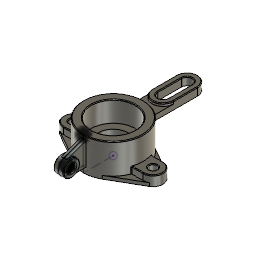
hw1 (Autodesk Fusion 360 design; units mm, degrees)
part number: 2026-08-05-10-36-34-167
Autodesk Fusion 360 part; units mm, degrees
sketch "스케치1" plane through (0, 0, 0) normal (0, 0, 1) x (1, 0, 0)
  circle A0 centre (0, 0) radius 45
  circle A1 centre (0, 0) radius 33
  circle A2 centre (0, 0) radius 22
  dimension "d3" = 90
  dimension "d9" = 66
  dimension "d10" = 44
  constraint concentric A0 A1
  constraint concentric A0 A2
  constraint coincident A0.centre A1.centre
  measures "d3" diameter of A0
  measures "d9" diameter of A1
  measures "d10" diameter of A2
sketch "스케치2" plane through (0, 0, 0) normal (0, 0, 1) x (1, 0, 0)
  line L0 (-8, 111) -> (-8, 75)
  arc A0 (-8, 75) -> (8, 75) centre (0, 75) ccw
  line L1 (8, 75) -> (8, 111)
  arc A1 (8, 111) -> (-8, 111) centre (0, 111) ccw
  line L2 (0, 111) -> (0, 75) construction
  line L3 (-16, 111) -> (-16, 75)
  arc A2 (-16, 75) -> (16, 75) centre (0, 75) ccw
  line L4 (16, 75) -> (16, 111)
  arc A3 (16, 111) -> (-16, 111) centre (0, 111) ccw
  line L5 (0, 111) -> (0, 75) construction
  line L6 (-16, 75) -> (-16, 42.0595)
  line L7 (16, 75) -> (16, 42.0595)
  circle A4 centre (0, 0) radius 45
  line L8 (0, 0) -> (0, 127) construction
  dimension "d15" = 16
  dimension "d16" = 32
  dimension "d17" = 36
  dimension "d18" = 75
  constraint tangent L0 A0
  constraint tangent A0 L1
  constraint parallel L0 L1
  constraint tangent L1 A1
  constraint tangent L0 A1
  constraint vertical L2
  constraint tangent L3 A2
  constraint tangent A2 L4
  constraint parallel L3 L4
  constraint tangent L4 A3
  constraint tangent L3 A3
  constraint parallel L1 L5
  constraint coincident A1.centre L2.start
  constraint coincident A0.centre L2.end
  constraint tangent A2 L6
  constraint tangent A2 L7
  constraint coincident L6.end A4
  constraint coincident L7.end A4
  constraint coincident A4.centre L8.start
  constraint midpoint A3 L8.end
  constraint vertical L8
  measures "d15" diameter of A0
  measures "d16" diameter of A2
  measures "d17" distance of A1.centre A0.centre
  measures "d18" distance of A0.centre A4.centre
extrude "돌출3" add sketch "스케치1" along normal blind 50 contours A0 makes body 1
extrude "돌출4" add sketch "스케치1" along normal blind 19 contours A1 bodies 1
extrude "돌출5" add sketch "스케치2" along normal blind 42 separate body contours L3 A2 L4 A3 makes body 2
extrude "돌출6" add sketch "스케치2" along normal blind 38 contours A2 L6 L7 A4 bodies 1 2
sketch "스케치3" plane through (0, 0, 0) normal (0, 0, 1) x (1, 0, 0)
  line L0 (-26, 36.7287) -> (-26, 127)
  line L1 (-26, 127) -> (26, 127)
  line L2 (26, 127) -> (26, 36.7287)
  circle A0 centre (0, 0) radius 45
  arc A1 (16, 111) -> (-16, 111) centre (0, 111) ccw
  line L3 (-16, 75) -> (-16, 42.0595)
  line L4 (16, 75) -> (16, 111)
  dimension "d26" = 10
  dimension "d27" = 10
  constraint vertical L0
  constraint perpendicular L0 L1
  constraint coincident L0.start A0
  constraint coincident L2.end A0
  constraint vertical L2
  constraint tangent L1 A1
  measures "d26" distance of L0 L3
  measures "d27" distance of L2 L4
extrude "돌출7" cut sketch "스케치3" along normal blind 30 contours L0 L1 L2 A0 bodies 1
sketch "스케치4" plane through (0, 0, 0) normal (0, 0, 1) x (1, 0, 0)
  line L0 (0, 0) -> (75, 0) construction
  circle A0 centre (60, 0) radius 6
  line L1 (42.4264, -15) -> (60, -15)
  line L2 (60, 15) -> (42.4264, 15)
  line L3 (60, -15) -> (60, 15) construction
  circle A1 centre (0, 0) radius 45
  arc A2 (60, -15) -> (60, 15) centre (60, 0) ccw
  line L4 (22.5, 38.9711) -> (67.5, 12.9904)
  line L5 (22.5, -38.9711) -> (67.5, -12.9904)
  dimension "d28" = 30
  dimension "d29" = 12
  dimension "d30" = 60
  constraint coincident L0.start A1.centre
  constraint horizontal L0
  constraint coincident A0.centre L0
  constraint coincident A0.centre A2.centre
  constraint horizontal L2
  constraint horizontal L1
  constraint coincident L1.end A2
  constraint coincident L2.start A2
  constraint perpendicular L0 L3
  constraint coincident A0.centre L3
  constraint coincident L1.end L3.start
  constraint coincident L2.start L3.end
  constraint coincident L2.end A1
  constraint coincident L1.start A1
  constraint tangent A2 L4
  constraint tangent A1 L4
  constraint coincident A1 L4.start
  constraint coincident A2 L4.end
  constraint tangent A2 L5
  constraint tangent A1 L5
  constraint coincident A1 L5.start
  constraint coincident A2 L5.end
  constraint coincident L0.end A2
  measures "d28" diameter of A2
  measures "d29" diameter of A0
  measures "d30" distance of A0.centre L0.start
extrude "돌출8" add sketch "스케치4" along normal blind 5 contours L2 A1 A2 L4 bodies 1
extrude "돌출9" add sketch "스케치4" along normal blind 5 contours L1 A1 A2 L5 bodies 1
extrude "돌출10" add sketch "스케치4" along normal blind 15 contours L1 L2 A1 A2 bodies 1
mirror "미러1" about plane through (0, 0, 0) normal (1, 0, 0) of "돌출9"
mirror "미러2" about plane through (0, 0, 0) normal (1, 0, 0) of "돌출10"
mirror "미러3" about plane through (0, 0, 0) normal (1, 0, 0) of "돌출8"
sketch "스케치5" plane through (0, 0, 0) normal (1, 0, 0) x (0, 1, 0)
  circle A0 centre (-70, 22) radius 12.5
  circle A1 centre (-70, 22) radius 7.5
  line L0 (-70, 9.5) -> (-45, 9.5)
  line L1 (-74.3101, 33.7334) -> (-45, 44.5)
  line L2 (0, 0) -> (-45, 0) construction
  line L3 (-45, 0) -> (-45, 9.5) construction
  line L4 (-45, 44.5) -> (-45, 50) construction
  line L5 (-45, 9.5) -> (-45, 44.5)
  dimension "d43" = 25
  dimension "d44" = 15
  dimension "d46" = 45
  dimension "d47" = 50
  dimension "d48" = 22
  dimension "d49" = 35
  dimension "d50" = 70
  constraint coincident A0.centre A1.centre
  constraint horizontal L0
  constraint tangent A0 L0
  constraint coincident A0 L0.start
  constraint coincident A0 L1.start
  constraint tangent A0 L1
  constraint coincident L2.start origin
  constraint horizontal L2
  constraint perpendicular L2 L3
  constraint coincident L1.end L3
  constraint parallel L3 L4
  measures "d43" diameter of A0
  measures "d44" diameter of A1
  measures "d46" distance of L2.start L2.end
  measures "d47" distance of L2.end L4.end
  measures "d48" vertical distance of L2.start A0.centre
  measures "d49" distance of L0 L1.end
  measures "d50" horizontal distance of L2.start A0.centre
extrude "돌출11" add sketch "스케치5" along normal mid plane 15 separate body contours A0 makes body 3
extrude "돌출12" add sketch "스케치5" along normal mid plane 8 separate body contours A0 L0 L1 L5 makes body 4
fillet "필렛1" radius 1 1 edges at (-42.4264, -15, 10) on bodies 1
fillet "필렛2" radius 1 1 edges at (-42.4264, 15, 10) on bodies 1
fillet "필렛3" radius 1 1 edges at (42.4264, 15, 10) on bodies 1
fillet "필렛4" radius 1 1 edges at (42.4264, -15, 10) on bodies 1
fillet "필렛5" radius 1 1 edges at (16, 42.0595, 34) on bodies 1
fillet "필렛6" radius 1 1 edges at (-16, 42.0595, 34) on bodies 1
fillet "필렛7" radius 1 1 edges at (-41.9547, -16.2727, 50) on bodies 1
fillet "필렛8" radius 1 1 edges at (-30.7668, 11.9333, 50) on bodies 1
fillet "필렛9" radius 1 4 edges at (16, 93, 42) (0, 127, 42) (-16, 93, 42) (0, 59, 42) on bodies 1
fillet "필렛10" radius 1 4 edges at (8, 93, 42) (0, 67, 42) (-8, 93, 42) (0, 119, 42) on bodies 1
fillet "필렛11" radius 1 5 edges at (42.5567, -15.1791, 15) (51.5639, -15, 15) (75, 0, 15) (51.5639, 15, 15) (42.5567, 15.1791, 15) on bodies 1
fillet "필렛12" radius 1 5 edges at (-42.5567, -15.1791, 15) (-51.5639, -15, 15) (-75, 0, 15) (-51.5639, 15, 15) (-42.5567, 15.1791, 15) on bodies 1
fillet "필렛13" radius 1 1 edges at (7.5, -81.6541, 17.4798) on bodies 3
fillet "필렛14" radius 1 1 edges at (-7.5, -81.6541, 26.5202) on bodies 3
fillet "필렛15" radius 1 1 edges at (-54.406, 2.1697, 0) on bodies 1
fillet "필렛16" radius 1 1 edges at (54.406, 2.1697, 0) on bodies 1
fillet "필렛17" radius 1 1 edges at (-54.406, 2.1697, 15) on bodies 1
fillet "필렛18" radius 1 1 edges at (54.406, 2.1697, 15) on bodies 1
